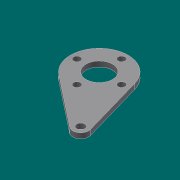
# Autodesk Inventor part: 長穴減速_ホーン_1_1
Saved by Autodesk Inventor 2016 (Build 200138000, 138)
## iProperties
Created: 2016-08-23
Part Number: 長穴減速_ホーン_1_1
Material: GFRP
Document SubType Name: Modeling
Designer: hiro
Mass: 1.66252 g
Surface Area: 12.9774 cm^2
Volume: 0.950012 cm^3
Density: 1.75 g/cm^3
Appearance: 滑らか - 淡い灰色
Author: hiro
Autodesk Inventor part; units mm, degrees
ref_plane "YZ Plane" through (0, 0, 0) normal (1, 0, 0) x (0, 1, 0)
ref_plane "XZ Plane" through (0, 0, 0) normal (0, 1, 0) x (-1, 0, 0)
ref_plane "XY Plane" through (0, 0, 0) normal (0, 0, 1) x (1, 0, 0)
derived "膝_基準フレーム_6_1.ipt"
sketch "スケッチ1" plane through (0, 0, 0) normal (0, 0, 1) x (1, 0, 0)
  line L0 (-16, 46.7205) -> (-16, 14.7205) construction
  line L1 (-16, 14.7205) -> (23.5, 14.7205) construction
  line L2 (-16, 46.7205) -> (23.5, 46.7205) construction
  line L3 (35.5, 41.3035) -> (35.5, 20.1375) construction
  arc A0 (35.5, 41.3035) -> (23.5, 46.7205) centre (23.5, 30.7205) ccw construction
  arc A1 (23.5, 14.7205) -> (35.5, 20.1375) centre (23.5, 30.7205) ccw construction
  circle A2 centre (23.5, 30.7205) radius 10.5 construction
  circle A3 centre (-22, 28.5) radius 1.55 construction
  circle A4 centre (10, 8.5) radius 5.05 construction
  line L4 (-22, 28.5) -> (78, 28.5) construction
  line L5 (10, 8.5) -> (110, 8.5) construction
  line L6 (10, 15.5) -> (110, 15.5) construction
  line L7 (10, 1.5) -> (110, 1.5) construction
  arc A5 (10, 15.5) -> (10, 1.5) centre (10, 8.5) ccw construction
  arc A6 (110, 1.5) -> (110, 15.5) centre (110, 8.5) ccw construction
  circle A7 centre (-22, 28.5) radius 5.5 construction
  line L8 (0, 0) -> (-46.0482, 0) construction
  arc A8 (110, -15.5) -> (110, -1.5) centre (110, -8.5) ccw construction
  line L9 (10, -1.5) -> (110, -1.5) construction
  line L10 (10, -8.5) -> (110, -8.5) construction
  line L11 (10, -15.5) -> (110, -15.5) construction
  line L12 (-22, -28.5) -> (78, -28.5) construction
  line L13 (35.5, -41.3035) -> (35.5, -20.1375) construction
  circle A9 centre (10, -8.5) radius 5.05 construction
  arc A10 (10, -1.5) -> (10, -15.5) centre (10, -8.5) ccw construction
  arc A11 (23.5, -46.7205) -> (35.5, -41.3035) centre (23.5, -30.7205) ccw construction
  arc A12 (35.5, -20.1375) -> (23.5, -14.7205) centre (23.5, -30.7205) ccw construction
  circle A13 centre (23.5, -30.7205) radius 10.5 construction
  line L14 (-16, -46.7205) -> (-16, -14.7205) construction
  line L15 (-16, -14.7205) -> (23.5, -14.7205) construction
  line L16 (-16, -46.7205) -> (23.5, -46.7205) construction
  circle A14 centre (-22, -28.5) radius 1.55 construction
  circle A15 centre (-22, -28.5) radius 5.5 construction
  line L17 (39.9042, 9.2519) -> (33.6649, 33.3521) construction
  line L18 (34.9944, 6.2689) -> (16.4805, 22.9118) construction
  arc A16 (34.9944, 6.2689) -> (39.9042, 9.2519) centre (37, 8.5) ccw construction
  arc A17 (33.6649, 33.3521) -> (16.4805, 22.9118) centre (23.5, 30.7205) ccw construction
  line L19 (37, 8.5) -> (23.5, 30.7205) construction
  line L20 (10, 8.5) -> (23.5, 30.7205) construction
  circle A18 centre (22.5, 44.2205) radius 1.35 construction
  circle A19 centre (22.5, 17.2205) radius 1.35 construction
  circle A20 centre (-4.5, 17.2205) radius 1.35 construction
  line L21 (22.5, 17.2205) -> (-4.5, 17.2205) construction
  line L22 (-4.5, 17.2205) -> (-4.5, 44.2205) construction
  line L23 (-4.5, 44.2205) -> (22.5, 44.2205) construction
  line L24 (22.5, 44.2205) -> (22.5, 17.2205) construction
  circle A21 centre (23.5, 30.7205) radius 11 construction
  circle A22 centre (-22, 28.5) radius 1.55 construction
  circle A23 centre (10, 8.5) radius 1.55 construction
  circle A24 centre (-4.5, 44.2205) radius 1.35 construction
  circle A25 centre (-22, -28.5) radius 1.55 construction
  circle A26 centre (-4.5, -44.2205) radius 1.35 construction
  circle A27 centre (-4.5, -17.2205) radius 1.35 construction
  circle A28 centre (22.5, -17.2205) radius 1.35 construction
  circle A29 centre (10, -8.5) radius 1.55 construction
  circle A30 centre (22.5, -44.2205) radius 1.35 construction
  circle A31 centre (23.5, -30.7205) radius 11 construction
  line L25 (-27.5, 28.5) -> (-27.5, -28.5) construction
  arc A32 (-25.1237, 33.0269) -> (-27.5, 28.5) centre (-22, 28.5) ccw construction
  line L26 (-25.1237, 33.0269) -> (-5.2788, 46.7205) construction
  line L27 (-5.2788, 46.7205) -> (-3.2946, 46.7205) construction
  line L28 (-3.2946, 46.7205) -> (14.8935, 23.87) construction
  circle A33 centre (-4.5, 44.2205) radius 2.5 construction
  arc A34 (14.8935, 23.87) -> (25, 19.8232) centre (23.5, 30.7205) ccw construction
  line L29 (25, 19.8232) -> (25, 14.3677) construction
  circle A35 centre (22.5, 17.2205) radius 2.5 construction
  line L30 (25, 14.3677) -> (25, 0.6427) construction
  line L31 (-25.1237, -33.0269) -> (-5.2788, -46.7205) construction
  arc A36 (-27.5, -28.5) -> (-25.1237, -33.0269) centre (-22, -28.5) ccw construction
  line L32 (-3.2946, -46.7205) -> (14.8935, -23.87) construction
  arc A37 (25, -19.8232) -> (14.8935, -23.87) centre (23.5, -30.7205) ccw construction
  line L33 (25, -19.8232) -> (25, -14.3677) construction
  line L34 (25, -14.3677) -> (25, 0.6427) construction
  line L35 (-5.2788, -46.7205) -> (-3.2946, -46.7205) construction
  circle A38 centre (23.5, 30.7205) radius 5.05
  circle A39 centre (37, 8.5) radius 1.55
  circle A40 centre (32, 30.7205) radius 1.35
  circle A41 centre (23.5, 39.2205) radius 1.35
  circle A42 centre (15, 30.7205) radius 1.35
  circle A43 centre (23.5, 22.2205) radius 1.35
  arc A44 (34.2023, 33.2623) -> (16.3125, 22.3934) centre (23.5, 30.7205) ccw
  line L36 (16.3125, 22.3934) -> (35.0398, 6.229)
  line L37 (34.2023, 33.2623) -> (39.9188, 9.1932)
  arc A45 (35.0398, 6.229) -> (39.9188, 9.1932) centre (37, 8.5) ccw
  circle A46 centre (10, 8.5) radius 5.6 construction
  circle A47 centre (-22, 28.5) radius 5.6 construction
  line L38 (23.5, 30.7205) -> (37, 52.941) construction
  circle A48 centre (23.5, 30.7205) radius 26 construction
  circle A49 centre (10, 8.5) radius 52 construction
  line L39 (23.5, 30.7205) -> (-2.4935, 30.1394) construction
  line L40 (10, 8.5) -> (-16, 53.5333) construction
  line L41 (-2.4935, 30.1394) -> (-16, 53.5333) construction
  line L42 (37, 8.5) -> (62, 8.5) construction
  point P0 (35.5, 30.7205)
  point P1 (35.5, -30.7205)
  point P2 (22.5, 30.7205)
  dimension "d7" = 10.1
  dimension "d15" = 3.1
  dimension "d17" = 2.7
  dimension "d27" = 8.5
  dimension "d31" = 360
  dimension "d35" = 11
  measures "d7" diameter of A38
  measures "d15" diameter of A39
  measures "d17" diameter of A40
  measures "d27" distance of A40.centre L38.start
  measures "d35" radius of A44
extrude "押し出し1" add sketch "スケッチ1" along normal blind 2
